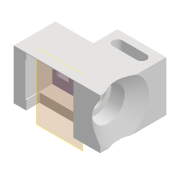
# Autodesk Inventor part: 30_Scanlens_Laseradaper_v0
Saved by Autodesk Inventor 2022 (Build 260153000, 153)
## iProperties
Created: 2022-12-16
Part Number: 30_Scanlens_Laseradaper_v0
Material: Generisch
Document SubType Name: Modeling
Designer: UC2
Density: 1 g/cm^3
Appearance: Vorgabe
Author: UC2
Autodesk Inventor part; units mm, degrees
ref_plane "YZ Plane" through (0, 0, 0) normal (1, 0, 0) x (0, 1, 0)
ref_plane "XZ Plane" through (0, 0, 0) normal (0, 1, 0) x (-1, 0, 0)
ref_plane "XY Plane" through (0, 0, 0) normal (0, 0, 1) x (1, 0, 0)
ref_plane "Arbeitsebene1" through (0, 0, 0) normal (0, 0, 1) x (1, 0, 0)
ref_plane "Arbeitsebene2" through (-2.35, 3.95, -7.1) normal (0, 0, -1) x (-1, 0, 0)
sketch "Skizze1" plane through (-2.35, 3.95, -7.1) normal (0, 0, -1) x (-1, 0, 0)
  line L0 (7.75, 3.25) -> (7.75, -3.25) projected
  line L1 (7.75, -3.25) -> (2.75, -3.25) projected
  line L2 (2.75, -3.25) -> (2.75, 3.25) projected
  line L3 (2.75, 3.25) -> (7.75, 3.25) projected
  line L4 (9.25, -6.8) -> (9.25, 6.8) projected
  line L5 (9.25, 6.8) -> (-9.25, 6.8) projected
  line L6 (-9.25, 6.8) -> (-9.25, -6.8) projected
  line L7 (-9.25, -6.8) -> (9.25, -6.8) projected
  line L8 (14.25, 9.8) -> (-21.25, 9.8)
  line L9 (-21.25, 9.8) -> (-21.25, -10.8)
  line L10 (-21.25, -10.8) -> (14.25, -10.8)
  line L11 (14.25, -10.8) -> (14.25, 9.8)
  point P0 (-2.35, -3.95)
  dimension "d0" = 5
  dimension "d1" = 3
  dimension "d2" = 4
  dimension "d3" = 12
  constraints: 8 end point, 2 parallel, 1 horizontal, 1 perpendicular
  measures "d0" distance between parallel lines of L11 L4
  measures "d1" distance between parallel lines of L5 L8
  measures "d2" distance between parallel lines of L10 L7
  measures "d3" distance between parallel lines of L9 L6
extrude "Extrusion1" add sketch "Skizze1" along normal blind 6 contours L7 L6 L5 L4 | L11 L10 L9 L8
sketch "Skizze2" plane through (-2.35, 3.95, -7.1) normal (0, 0, 1) x (1, 0, 0)
  line L0 (-9.25, -6.8) -> (-9.25, 6.8) projected
  line L1 (9.25, -6.8) -> (-9.25, -6.8) projected
  line L2 (9.25, 6.8) -> (9.25, -6.8) projected
  line L3 (-9.25, 6.8) -> (9.25, 6.8) projected
  line L4 (9.55, 7.1) -> (9.55, -7.1)
  line L5 (9.55, -7.1) -> (-9.55, -7.1)
  line L6 (-9.55, -7.1) -> (-9.55, 7.1)
  line L7 (-9.55, 7.1) -> (9.55, 7.1)
  line L8 (21.25, 9.8) -> (21.25, -10.8) projected
  line L9 (-14.25, 9.8) -> (21.25, 9.8) projected
  line L10 (-14.25, -10.8) -> (-14.25, 9.8) projected
  line L11 (21.25, -10.8) -> (-14.25, -10.8) projected
  line L12 (-7.75, 3.25) -> (-7.75, -3.25) projected
  line L13 (-2.75, 3.25) -> (-7.75, 3.25) projected
  line L14 (-2.75, -3.25) -> (-2.75, 3.25) projected
  line L15 (-7.75, -3.25) -> (-2.75, -3.25) projected
  point P0 (2.35, -3.95)
  dimension "d6" = 0.3
  constraints: 8 end point, 3 other
  measures "d6" distance between parallel lines of L3 L7
ref_plane "Arbeitsebene3" through (-10.5, -12.5, -1.5) normal (0, 0, -1) x (0, 1, 0)
extrude "Extrusion2" add sketch "Skizze2" along normal up to surface (5.6 mm away) contours L8 L11 L10 L9
sketch "Skizze3" plane through (-16.6, 13.75, -1.5) normal (0, 0, 1) x (1, 0, 0)
  line L0 (23.5, -26.25) -> (23.5, -1.25) projected
  line L1 (23.5, -1.25) -> (6.1, -1.25) projected
  line L2 (6.1, -1.25) -> (6.1, -26.25) projected
  line L3 (6.1, -26.25) -> (23.5, -26.25) projected
  line L4 (24.5, -27.25) -> (24.5, -0.25)
  line L5 (24.5, -0.25) -> (5.1, -0.25)
  line L6 (5.1, -0.25) -> (5.1, -27.25)
  line L7 (5.1, -27.25) -> (24.5, -27.25)
  line L8 (4.7, -2.7) -> (23.8, -2.7) projected
  line L9 (23.8, -2.7) -> (23.8, -16.9) projected
  line L10 (23.8, -16.9) -> (4.7, -16.9) projected
  line L11 (4.7, -16.9) -> (4.7, -2.7) projected
  line L12 (35.5, 0) -> (0, 0) projected
  line L13 (0, 0) -> (0, -20.6) projected
  line L14 (0, -20.6) -> (35.5, -20.6) projected
  line L15 (35.5, -20.6) -> (35.5, 0) projected
  point P0 (16.6, -13.75)
  point P1 (24.5, -20.6)
  point P2 (5.1, -20.6)
  point P3 (5.1, -16.9)
  point P4 (5.1, -2.7)
  dimension "d9" = 1
  constraints: 8 end point, 3 other
  measures "d9" distance between parallel lines of L3 L7
extrude "Extrusion3" add sketch "Skizze3" along normal blind 5.5 contours L4 L5 L6 L8 L11 L10 L14 L13 L12 L15
sketch "Skizze4" plane through (18.9, -6.85, -13.1) normal (1, 0, 0) x (0, 0, -1)
  circle A0 centre (-8.8, 10.8) radius 6.75
  circle A1 centre (-8.8, 10.8) radius 6.5405 projected
  point P0 (-13.1, 6.85)
  dimension "d30" = 13.5
  constraints: 1 centre point, 1 coincident
  measures "d30" diameter of A0
extrude "Extrusion4" cut sketch "Skizze4" against normal blind 10.5 contours A0 | A1
sketch "Skizze5" plane through (8.4, -6.85, -13.1) normal (1, 0, 0) x (0, 0, -1)
  circle A0 centre (-8.8, 10.8) radius 4.5085 projected
  point P0 (-13.1, 6.85)
extrude "Extrusion5" cut sketch "Skizze5" against normal blind 6
sketch "Skizze6" plane through (-16.6, -6.85, -13.1) normal (0, -1, 0) x (1, 0, 0)
  line L0 (0, 17.1) -> (0, 0) projected
  line L1 (35.5, 0) -> (0, 0) projected
  line L2 (35.5, 17.1) -> (35.5, 0) projected
  line L3 (24.5, 17.1) -> (35.5, 17.1) projected
  line L4 (24.5, 11.6) -> (24.5, 17.1) projected
  line L5 (5.1, 11.6) -> (24.5, 11.6) projected
  line L6 (5.1, 11.6) -> (5.1, 17.1) projected
  line L7 (0, 17.1) -> (5.1, 17.1) projected
  line L8 (11.5, 6) -> (11.5, 0) projected
  line L9 (35.5, 0) -> (15.5, 0)
  line L10 (15.5, 0) -> (15.5, -10)
  line L11 (15.5, -10) -> (35.5, -10)
  line L12 (35.5, -10) -> (35.5, 0)
  line L13 (30.4199, -5) -> (20.5801, -5) construction
  line L14 (30.4199, -3) -> (20.5801, -3)
  line L15 (20.5801, -7) -> (30.4199, -7)
  arc A0 (30.4199, -7) -> (30.4199, -3) centre (30.4199, -5) ccw
  arc A1 (20.5801, -3) -> (20.5801, -7) centre (20.5801, -5) ccw
  point P0 (16.6, 13.1)
  point P1 (25.5, -5)
  dimension "d19" = 20
  dimension "d20" = 10
  dimension "d21" = 4
  constraints: 16 end point, 4 point on circle, 4 tangent, 3 parallel, 2 centre point, 2 horizontal, 1 midpoint, 1 perpendicular
  measures "d19" distance of L11.end L10.end
  measures "d20" distance of L10.end L9.end
  measures "d21" diameter of A1
extrude "Extrusion6" add sketch "Skizze6" against normal up to surface (20.6 mm away) contours L1 L12 L11 L10
chamfer "Fase1" distance 5 angle 45 1 edges at (18.9, 3.95, 2.45)
chamfer "Fase2" distance 4 angle 45 4 edges at (-7.6, 0.7, -13.1) (-10.1, 3.95, -13.1) (-7.6, 7.2, -13.1) (-5.1, 3.95, -13.1)
